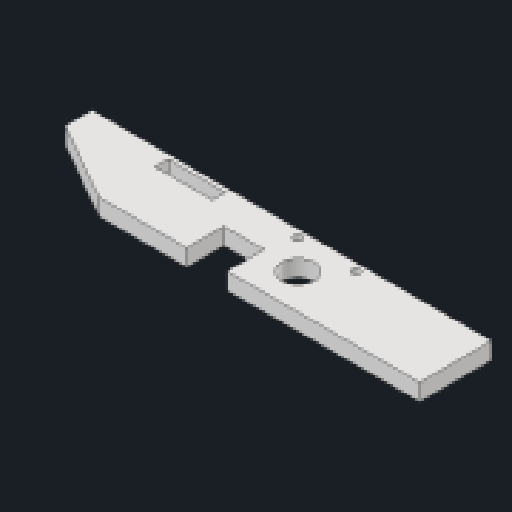
# Autodesk Inventor part: right_hold
Saved by Autodesk Inventor 2023 (Build 270158000, 158)
## iProperties
Created: 2024-04-29
Part Number: right_hold
Material: Generic
Document SubType Name: Modeling
Designer: szymo
Density: 1 g/cm^3
Appearance: Default
Mass: 29.78 g
Surface Area: 120.238 cm^2
Volume: 29.78 cm^3
Author: szymo
Autodesk Inventor part; units mm, degrees
ref_plane "YZ Plane" through (0, 0, 0) normal (1, 0, 0) x (0, 1, 0)
ref_plane "XZ Plane" through (0, 0, 0) normal (0, 1, 0) x (-1, 0, 0)
ref_plane "XY Plane" through (0, 0, 0) normal (0, 0, 1) x (1, 0, 0)
sketch "Sketch1" plane through (0, 0, 0) normal (0, 0, 1) x (1, 0, 0)
  line L0 (91, -34) -> (91, 34) projected
  line L1 (91, 34) -> (41, 34) projected
  line L2 (41, 34) -> (41, 89) projected
  line L3 (41, 89) -> (-91, 89) projected
  line L4 (-91, 89) -> (-91, -89) projected
  line L5 (-91, -89) -> (41, -89) projected
  line L6 (41, -89) -> (41, -34) projected
  line L7 (41, -34) -> (91, -34) projected
  line L8 (70, 27) -> (62, 27) projected
  line L9 (91, 34) -> (-87, 34)
  line L10 (-87, 34) -> (-87, 27)
  line L11 (-87, 27) -> (91, 27)
  line L12 (91, 27) -> (91, 34)
  circle A0 centre (-83, 21.5) radius 1.2295 projected
  circle A1 centre (-83, -64.5) radius 1.2295 projected
  circle A2 centre (-83, -21.5) radius 1.2295 projected
  circle A3 centre (-83, 64.5) radius 1.2295 projected
  line L13 (-85, -72) -> (-76, -72) projected
  line L14 (-76, -72) -> (-76, -57) projected
  line L15 (-76, -57) -> (-85, -57) projected
  arc A4 (-87, -55) -> (-85, -57) centre (-85, -55) ccw projected
  line L16 (-87, -55) -> (-87, -31) projected
  arc A5 (-85, -29) -> (-87, -31) centre (-85, -31) ccw projected
  line L17 (-85, -29) -> (-76, -29) projected
  line L18 (-76, -29) -> (-76, -14) projected
  line L19 (-76, -14) -> (-85, -14) projected
  arc A6 (-87, -12) -> (-85, -14) centre (-85, -12) ccw projected
  line L20 (-87, -12) -> (-87, 12) projected
  arc A7 (-85, 14) -> (-87, 12) centre (-85, 12) ccw projected
  line L21 (-85, 14) -> (-76, 14) projected
  line L22 (-76, 14) -> (-76, 29) projected
  line L23 (-76, 29) -> (-85, 29) projected
  arc A8 (-87, 31) -> (-85, 29) centre (-85, 31) ccw projected
  line L24 (-87, 31) -> (-87, 55) projected
  arc A9 (-85, 57) -> (-87, 55) centre (-85, 55) ccw projected
  line L25 (-85, 57) -> (-76, 57) projected
  line L26 (-76, 57) -> (-76, 72) projected
  line L27 (-76, 72) -> (-85, 72) projected
  arc A10 (-87, 74) -> (-85, 72) centre (-85, 74) ccw projected
  line L28 (-87, 74) -> (-87, 89) projected
  line L29 (-91, 89) -> (-87, 89) projected
  line L30 (-91, -89) -> (-91, 89) projected
  line L31 (-91, -89) -> (-87, -89) projected
  line L32 (-87, -89) -> (-87, -74) projected
  arc A11 (-85, -72) -> (-87, -74) centre (-85, -74) ccw projected
  line L33 (-91, 89.5) -> (-86.5, 89.5)
  line L34 (-86.5, 89.5) -> (-86.5, 74)
  arc A12 (-86.5, 74) -> (-85, 72.5) centre (-85, 74) ccw
  line L35 (-85, 72.5) -> (-75.5, 72.5)
  line L36 (-75.5, 72.5) -> (-75.5, 56.5)
  line L37 (-75.5, 56.5) -> (-85, 56.5)
  arc A13 (-85, 56.5) -> (-86.5, 55) centre (-85, 55) ccw
  line L38 (-86.5, 55) -> (-86.5, 31)
  arc A14 (-86.5, 31) -> (-85, 29.5) centre (-85, 31) ccw
  line L39 (-85, 29.5) -> (-75.5, 29.5)
  line L40 (-75.5, 29.5) -> (-75.5, 13.5)
  line L41 (-75.5, 13.5) -> (-85, 13.5)
  arc A15 (-85, 13.5) -> (-86.5, 12) centre (-85, 12) ccw
  line L42 (-86.5, 12) -> (-86.5, -12)
  arc A16 (-86.5, -12) -> (-85, -13.5) centre (-85, -12) ccw
  line L43 (-85, -13.5) -> (-75.5, -13.5)
  line L44 (-75.5, -13.5) -> (-75.5, -29.5)
  line L45 (-75.5, -29.5) -> (-85, -29.5)
  arc A17 (-85, -29.5) -> (-86.5, -31) centre (-85, -31) ccw
  line L46 (-86.5, -31) -> (-86.5, -55)
  arc A18 (-86.5, -55) -> (-85, -56.5) centre (-85, -55) ccw
  line L47 (-85, -56.5) -> (-75.5, -56.5)
  line L48 (-75.5, -56.5) -> (-75.5, -72.5)
  line L49 (-75.5, -72.5) -> (-85, -72.5)
  arc A19 (-85, -72.5) -> (-86.5, -74) centre (-85, -74) ccw
  line L50 (-86.5, -74) -> (-86.5, -89.5)
  line L51 (-86.5, -89.5) -> (-91, -89.5)
  line L52 (-86.5, 31) -> (-75.5, 31)
  line L53 (-75.5, 31) -> (-75.5, 29.5)
  line L54 (-75.5, 31) -> (-75.5, 34)
  point P0 (0, 0)
  point P1 (-75.5, 27)
  point P2 (-86.5, 34)
  dimension "d6" = 0.5
  constraints: 52 end point, 16 point on circle, 8 centre point, 3 perpendicular, 2 collinear, 2 horizontal, 2 parallel, 1 point on line, 26 other
  measures "d6" distance between parallel lines of L22 L40
extrude "Extrusion1" add sketch "Sketch1" along normal blind 30 contours L11 L8 L40 L53 L54 L9 L1 L0
sketch "Sketch3" plane through (-86.5, 34, 0) normal (0, 1, 0) x (1, 0, 0)
  line L0 (-0.5, -4.5) -> (-0.5, 0) projected
  line L1 (-0.5, 0) -> (-4.5, 0) projected
  line L2 (-4.5, 0) -> (-4.5, 3.5) projected
  line L3 (-4.5, 3.5) -> (-18.5, 3.5) projected
  line L4 (-18.5, 3.5) -> (-4.5, -5.5) projected
  line L5 (-4.5, -5.5) -> (-4.5, -4.5) projected
  line L6 (-4.5, -4.5) -> (-0.5, -4.5) projected
  line L7 (-0.5, -4.5) -> (50.0525, -33.6865)
  line L8 (177.5, 0) -> (11, 0) projected
  line L9 (177.5, -30) -> (11, -30) projected
  line L10 (177.5, 0) -> (177.5, -30) projected
  line L11 (11, 0) -> (11, -30) projected
  point P0 (86.5, 0)
  point P1 (43.6673, -30)
  point P2 (11, -11.1395)
  dimension "d7" = 30
  constraints: 2 end point
  measures "d7" angle of L7 L6
extrude "Extrusion4" cut sketch "Sketch3" against normal blind 30 contours L7 L9 L11
sketch "Sketch5" plane through (-75.5, 27, 0) normal (0, -1, 0) x (1, 0, 0)
  line L0 (56.5, 7.0341) -> (57.5, 7.0341) projected
  line L1 (34.5, 7.0341) -> (56.5, 7.0341) projected
  line L2 (33.5, 7.0341) -> (33.5, 6.6226)
  line L3 (33.5, 6.6226) -> (9.5, 6.6226)
  line L4 (9.5, 6.6226) -> (9.5, 7.0341)
  line L5 (9.5, 7.0341) -> (33.5, 7.0341)
  line L6 (64.5, 7.0341) -> (64.5, 6.6226)
  line L7 (64.5, 6.6226) -> (57.5, 6.6226)
  line L8 (57.5, 6.6226) -> (57.5, 7.0341)
  line L9 (57.5, 7.0341) -> (64.5, 7.0341)
  line L10 (9.5, 2) -> (9.5, 2.6226)
  line L11 (9.5, 2.6226) -> (64.5, 2.6226)
  line L12 (64.5, 2.6226) -> (64.5, 2)
  line L13 (64.5, 2) -> (9.5, 2)
  line L14 (9.5, 7.0341) -> (64.5, 7.0341)
  line L15 (64.5, 7.0341) -> (64.5, 2)
  line L16 (64.5, 2) -> (9.5, 2)
  line L17 (9.5, 2) -> (9.5, 7.0341)
  line L18 (9.2, 7.3341) -> (64.8, 7.3341)
  line L19 (64.8, 7.3341) -> (64.8, 1.9)
  line L20 (64.8, 1.9) -> (9.2, 1.9)
  line L21 (9.2, 1.9) -> (9.2, 7.3341)
  point P0 (75.5, 0)
  dimension "d19" = 0.3
  dimension "d20" = 0.3
  dimension "d21" = 0.1
  dimension "d22" = 0.3
  constraints: 40 end point, 8 horizontal, 6 vertical, 4 parallel, 2 perpendicular, 11 other
  measures "d19" distance between parallel lines of L21 L17
  measures "d20" distance between parallel lines of L19 L15
  measures "d21" distance between parallel lines of L13 L20
  measures "d22" distance between parallel lines of L18 L1
extrude "Extrusion6" cut sketch "Sketch5" against normal blind 0.7 contours L0 L8 L7 L15 L11 L17 L3 L2 L14 L1 | L9 L6 L7 L8 | L2 L3 L4 L5 | L12 L13 L10 L11 | L18 L19 L20 L21
sketch "Sketch6" plane through (-75.5, 27, 0) normal (0, -1, 0) x (1, 0, 0)
  line L0 (33.5, 7.0341) -> (34.5, 7.0341) projected
  line L1 (34.5, 7.0341) -> (56.5, 7.0341) projected
  line L2 (56.5, 7.0341) -> (57.5, 7.0341) projected
  line L3 (64.8, 1.9) -> (9.2, 1.9) projected
  line L4 (64.8, 7.3341) -> (64.8, 1.9) projected
  line L5 (9.2, 7.3341) -> (64.8, 7.3341) projected
  line L6 (9.2, 1.9) -> (9.2, 7.3341) projected
  line L7 (33.5, 7.3341) -> (57.5, 7.3341)
  line L8 (57.5, 7.3341) -> (57.5, 1.9)
  line L9 (57.5, 1.9) -> (33.5, 1.9)
  line L10 (33.5, 1.9) -> (33.5, 7.3341)
  point P0 (75.5, 0)
  constraints: 8 end point, 4 point on line, 2 parallel, 1 horizontal, 1 perpendicular
extrude "Extrusion7" cut sketch "Sketch6" against normal up to next contours L10 L5 L8 L2 L1 L0 | L0 L1 L2 L8 L3 L10
sketch "Sketch7" plane through (0, 0, 30) normal (0, 0, 1) x (1, 0, 0)
  line L0 (10.25, -34) -> (10.25, 34) projected
  line L1 (10.25, 34) -> (-5.75, 34) projected
  line L2 (-5.75, -34) -> (-5.75, 34) projected
  line L3 (10.25, -34) -> (-5.75, -34) projected
  line L4 (-42.8327, 27) -> (91, 27) projected
  line L5 (10.25, 34) -> (-5.75, 34)
  line L6 (-5.75, 34) -> (-5.75, 27)
  line L7 (-5.75, 27) -> (10.25, 27)
  line L8 (10.25, 27) -> (10.25, 34)
  line L9 (10.65, 34) -> (-6.15, 34)
  line L10 (-6.15, 34) -> (-6.15, 27)
  line L11 (-6.15, 27) -> (10.65, 27)
  line L12 (10.65, 27) -> (10.65, 34)
  point P0 (0, 0)
  dimension "d27" = 0.4
  dimension "d28" = 0.4
  constraints: 16 end point, 4 parallel, 4 point on line, 2 horizontal, 2 perpendicular
  measures "d27" distance between parallel lines of L12 L0
  measures "d28" distance between parallel lines of L2 L10
extrude "Extrusion8" cut sketch "Sketch7" against normal blind 15.5 contours L4 L2 L1 L0 | L0 L9 L12 L4 | L4 L10 L9 L2
sketch "Sketch8" plane through (-75.5, 27, 0) normal (0, -1, 0) x (1, 0, 0)
  circle A0 centre (89, 3.25) radius 1.8 projected
  circle A1 centre (113.25, 3.25) radius 1.8 projected
  point P0 (75.5, 0)
  constraints: 2 coincident
hole "Hole1" at (13.5, 27, 3.25) at (37.75, 27, 3.25) direction (0, 1, 0) diameter 3.6 end through all countersink diameter 6.5 countersink angle 90 clearance for "Countersunk Flat Head Screw ISO 2009/7046" size "M3" standard "ISO"
sketch "Sketch9" plane through (91, 27, 0) normal (0, -1, 0) x (1, 0, 0)
  arc A0 (-67.8175, 18.3693) -> (-69.7313, 19.2694) centre (-70.7618, 14.5935) ccw projected
  arc A1 (-69.7313, 19.2694) -> (-70.2869, 18.54) centre (-65.375, 15.375) ccw projected
  arc A2 (-70.2869, 18.54) -> (-68.9106, 16.9341) centre (-66.053, 20.7758) ccw projected
  arc A3 (-68.9106, 16.9341) -> (-69.111, 16.3618) centre (-65.375, 15.375) ccw projected
  arc A4 (-69.111, 16.3618) -> (-71.1884, 15.965) centre (-69.2737, 11.5765) ccw projected
  arc A5 (-71.1884, 15.965) -> (-71.2091, 15.0484) centre (-65.375, 15.375) ccw projected
  arc A6 (-71.2091, 15.0484) -> (-69.1518, 14.5581) centre (-69.098, 19.3459) ccw projected
  arc A7 (-69.1518, 14.5581) -> (-68.9775, 13.9774) centre (-65.375, 15.375) ccw projected
  arc A8 (-68.9775, 13.9774) -> (-70.425, 12.4353) centre (-66.2964, 10.0103) ccw projected
  arc A9 (-70.425, 12.4353) -> (-69.9029, 11.6815) centre (-65.375, 15.375) ccw projected
  arc A10 (-69.9029, 11.6815) -> (-67.9503, 12.4942) centre (-70.721, 16.3992) ccw projected
  arc A11 (-67.9503, 12.4942) -> (-67.468, 12.1268) centre (-65.375, 15.375) ccw projected
  arc A12 (-67.468, 12.1268) -> (-67.7326, 10.0285) centre (-62.9672, 10.4933) ccw projected
  arc A13 (-67.7326, 10.0285) -> (-66.8672, 9.7255) centre (-65.375, 15.375) ccw projected
  arc A14 (-66.8672, 9.7255) -> (-65.7652, 11.5306) centre (-70.302, 13.0613) ccw projected
  arc A15 (-65.7652, 11.5306) -> (-65.159, 11.5169) centre (-65.375, 15.375) ccw projected
  arc A16 (-65.159, 11.5169) -> (-64.1397, 9.6638) centre (-60.5576, 12.8409) ccw projected
  arc A17 (-64.1397, 9.6638) -> (-63.2615, 9.9273) centre (-65.375, 15.375) ccw projected
  arc A18 (-63.2615, 9.9273) -> (-63.431, 12.0355) centre (-68.0011, 10.6071) ccw projected
  arc A19 (-63.431, 12.0355) -> (-62.9325, 12.3807) centre (-65.375, 15.375) ccw projected
  arc A20 (-62.9325, 12.3807) -> (-61.0187, 11.4806) centre (-59.9882, 16.1565) ccw projected
  arc A21 (-61.0187, 11.4806) -> (-60.4631, 12.21) centre (-65.375, 15.375) ccw projected
  arc A22 (-60.4631, 12.21) -> (-61.8394, 13.8159) centre (-64.697, 9.9742) ccw projected
  arc A23 (-61.8394, 13.8159) -> (-61.639, 14.3882) centre (-65.375, 15.375) ccw projected
  arc A24 (-61.639, 14.3882) -> (-59.5616, 14.785) centre (-61.4763, 19.1735) ccw projected
  arc A25 (-59.5616, 14.785) -> (-59.5409, 15.7016) centre (-65.375, 15.375) ccw projected
  arc A26 (-59.5409, 15.7016) -> (-61.5982, 16.1919) centre (-61.652, 11.4041) ccw projected
  arc A27 (-61.5982, 16.1919) -> (-61.7725, 16.7726) centre (-65.375, 15.375) ccw projected
  arc A28 (-61.7725, 16.7726) -> (-60.325, 18.3147) centre (-64.4536, 20.7397) ccw projected
  arc A29 (-60.325, 18.3147) -> (-60.8471, 19.0685) centre (-65.375, 15.375) ccw projected
  arc A30 (-60.8471, 19.0685) -> (-62.7997, 18.2558) centre (-60.029, 14.3508) ccw projected
  arc A31 (-62.7997, 18.2558) -> (-63.282, 18.6232) centre (-65.375, 15.375) ccw projected
  arc A32 (-63.282, 18.6232) -> (-63.0174, 20.7215) centre (-67.7828, 20.2567) ccw projected
  arc A33 (-63.0174, 20.7215) -> (-63.8828, 21.0245) centre (-65.375, 15.375) ccw projected
  arc A34 (-63.8828, 21.0245) -> (-64.9848, 19.2194) centre (-60.448, 17.6887) ccw projected
  arc A35 (-64.9848, 19.2194) -> (-65.591, 19.2331) centre (-65.375, 15.375) ccw projected
  arc A36 (-65.591, 19.2331) -> (-66.6103, 21.0862) centre (-70.1924, 17.9091) ccw projected
  arc A37 (-66.6103, 21.0862) -> (-67.4885, 20.8227) centre (-65.375, 15.375) ccw projected
  arc A38 (-67.4885, 20.8227) -> (-67.319, 18.7145) centre (-62.7489, 20.1429) ccw projected
  arc A39 (-67.319, 18.7145) -> (-67.8175, 18.3693) centre (-65.375, 15.375) ccw projected
  circle A40 centre (-65.375, 15.375) radius 5.8433
  circle A41 centre (-65.375, 15.375) radius 6.8433
  circle A42 centre (-25, 8.5) radius 5.5 projected
  point P0 (-91, 0)
  dimension "d38" = 1
  constraints: 2 centre point, 1 coincident
  measures "d38" radial gap between concentric circles of A40 A41
extrude "Extrusion9" cut sketch "Sketch9" against normal up to next contours A39 A38 A37 A36 A35 A34 A33 A32 A31 A30 A29 A28 A27 A26 A25 A24 A23 A22 A21 A20 A19 A18 A17 A16 A15 A14 A13 A12 A11 A10 A9 A8 A7 A6 A5 A4 A3 A2 A1 A0 | A0 A40 A38 A39 | A2 A3 A4 A40 | A40 A34 A35 A36 | A6 A7 A8 A40 | A40 A30 A31 A32 | A10 A11 A12 A40 | A40 A26 A27 A28 | A14 A15 A16 A40 | A18 A19 A20 A40 | A40 A22 A23 A24 | A41
body "Solid1"
